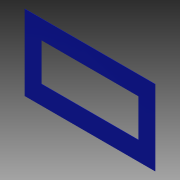
# Autodesk Inventor part: GE-13011B
Saved by Autodesk Inventor 2013 (Build 170138000, 138)
## iProperties
Created: 2013-01-04
Part Number: GE-13011B
Material: Polyethylene, High Density
Document SubType Name: Modeling
Designer: Phillip
Density: 1 g/cm^3
Author: Phillip
Autodesk Inventor part; units mm, degrees
ref_plane "YZ Plane" through (0, 0, 0) normal (1, 0, 0) x (0, 1, 0)
ref_plane "XZ Plane" through (0, 0, 0) normal (0, 1, 0) x (-1, 0, 0)
ref_plane "XY Plane" through (0, 0, 0) normal (0, 0, 1) x (1, 0, 0)
sketch "Sketch1" plane through (0, 0, 0) normal (0, 0, 1) x (1, 0, 0)
  line L0 (-920.75, -533.4) -> (920.75, -533.4)
  line L1 (920.75, -533.4) -> (920.75, 533.4)
  line L2 (920.75, 533.4) -> (-920.75, 533.4)
  line L3 (-920.75, 533.4) -> (-920.75, -533.4)
  line L4 (-920.75, -533.4) -> (920.75, 533.4) construction
  line L5 (920.75, -533.4) -> (-920.75, 533.4) construction
  point P0 (0, 0)
  dimension "d0" = 1841.5
  dimension "d1" = 1066.8
  constraints: 12 end point, 2 midpoint, 2 parallel, 1 horizontal, 1 perpendicular
  measures "d0" distance of L2.end L1.end
  measures "d1" distance of L1.end L0.end
extrude "Extrusion1" add sketch "Sketch1" against normal blind 3.175
sketch "Sketch2" plane through (0, 0, 0) normal (0, 0, 1) x (1, 0, 0)
  line L0 (-920.75, -533.4) -> (920.75, -533.4) projected
  line L1 (920.75, -533.4) -> (920.75, 533.4) projected
  line L2 (920.75, 533.4) -> (-920.75, 533.4) projected
  line L3 (-920.75, 533.4) -> (-920.75, -533.4) projected
  line L4 (-685.8, -266.7) -> (685.8, -266.7)
  line L5 (685.8, -266.7) -> (685.8, 266.7)
  line L6 (685.8, 266.7) -> (-685.8, 266.7)
  line L7 (-685.8, 266.7) -> (-685.8, -266.7)
  point P0 (0, 0)
  dimension "d4" = 234.95
  dimension "d5" = 266.7
  dimension "d6" = 234.95
  dimension "d7" = 266.7
  constraints: 8 end point, 2 parallel, 1 horizontal, 1 perpendicular
  measures "d4" distance between parallel lines of L7 L3
  measures "d5" distance between parallel lines of L2 L6
  measures "d6" distance between parallel lines of L1 L5
  measures "d7" distance between parallel lines of L0 L4
extrude "Extrusion2" cut sketch "Sketch2" against normal through all contours L7 L6 L5 L4
body "Solid1"
